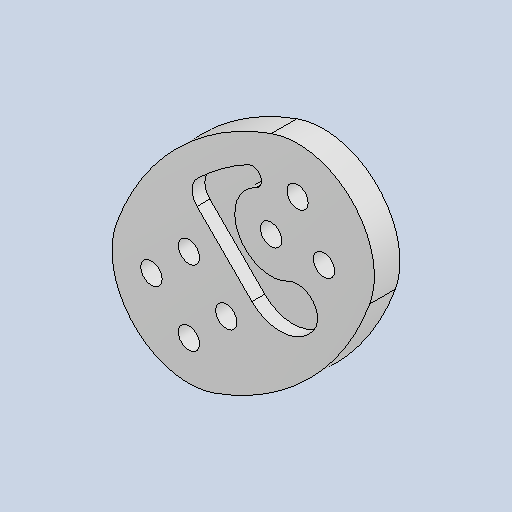
# Autodesk Inventor part: 駆動節
Saved by Autodesk Inventor 2023 (Build 270158000, 158)
## iProperties
Created: 2022-01-08
Part Number: 駆動節
Material: Aluminum 2014-T6
Document SubType Name: Modeling
Designer: acps
Density: 2.78927 g/cm^3
Appearance: Satin
Author: acps
Autodesk Inventor part; units mm, degrees
ref_plane "YZ Plane" through (0, 0, 0) normal (1, 0, 0) x (0, 1, 0)
ref_plane "XZ Plane" through (0, 0, 0) normal (0, 1, 0) x (-1, 0, 0)
ref_plane "XY Plane" through (0, 0, 0) normal (0, 0, 1) x (1, 0, 0)
sketch "Sketch2" plane through (0, 0, 0) normal (0, 0, 1) x (1, 0, 0)
  line L0 (-12.7279, -12.7279) -> (0, 0) construction
  line L1 (-12.7279, -12.7279) -> (-7.4558, -12.7279) construction
  line L2 (-12.7279, -12.7279) -> (0, 0) construction
  line L3 (-17.252, -29.9799) -> (-9.2664, -21.9943) construction
  line L4 (-2.9446, 9.7833) -> (-10.9302, 1.7977) construction
  arc A0 (-21.1882, -9.6582) -> (-9.6582, -21.1882) centre (-12.7279, -12.7279) ccw
  arc A1 (8.4603, -3.0697) -> (-3.0697, 8.4603) centre (0, 0) ccw
  circle A2 centre (-8.3439, -12.7279) radius 1.25
  circle A3 centre (-8.3439, -12.7279) radius 3.1 construction
  circle A4 centre (-12.7279, -8.3439) radius 1.25
  circle A5 centre (-12.7279, -8.3439) radius 3.1 construction
  circle A6 centre (-17.112, -12.7279) radius 1.25
  circle A7 centre (-17.112, -12.7279) radius 3.1 construction
  circle A8 centre (-12.7279, -17.112) radius 1.25
  circle A9 centre (-12.7279, -17.112) radius 3.1 construction
  circle A10 centre (-3.1, -1.7898) radius 1.25
  circle A11 centre (-3.1, -1.7898) radius 3.1 construction
  circle A12 centre (3.1, -1.7898) radius 3.1 construction
  circle A13 centre (3.1, -1.7898) radius 1.25
  circle A14 centre (0, 3.5796) radius 3.1 construction
  circle A15 centre (0, 3.5796) radius 1.25
  arc A16 (-9.6582, -21.1882) -> (8.4603, -3.0697) centre (-19.9758, 7.2478) ccw
  line L5 (1.4142, -14.1421) -> (-6.364, -6.364) construction
  arc A17 (-3.0697, 8.4603) -> (-21.1882, -9.6582) centre (7.2478, -19.9758) ccw
  point P0 (-6.364, -6.364)
  dimension "d34" = 18
  dimension "d35" = 9
  dimension "d36" = 2.5
  dimension "d37" = 6.2
  dimension "d38" = 360
  dimension "d39" = 2.5
  dimension "d40" = 6.2
  dimension "d41" = 360
  dimension "d42" = 11
  dimension "d43" = 45
  constraints: 18 centre point, 14 end point, 9 point on circle, 8 coincident, 8 tangent, 3 symmetric about line, 2 midpoint, 1 horizontal, 1 horizontal alignment, 1 parallel, 1 perpendicular, 1 vertical alignment, 31 other
  measures "d34" distance of L0.start L0.end
  measures "d35" radius of A1
  measures "d36" diameter of A2
  measures "d37" diameter of A3
  measures "d39" diameter of A10
  measures "d40" diameter of A11
  measures "d42" distance of L5.start L5.end
  measures "d43" angle of L1 L0
extrude "Extrusion2" add sketch "Sketch2" along normal blind 3
sketch "Sketch3" plane through (0, 0, 3) normal (0, 0, 1) x (1, 0, 0)
  circle A0 centre (-12.7279, -8.3439) radius 1.25 projected
  circle A1 centre (-8.3439, -12.7279) radius 1.25 projected
  arc A2 (-3.0697, 8.4603) -> (-21.1882, -9.6582) centre (7.2478, -19.9758) ccw projected
  arc A3 (-9.6582, -21.1882) -> (8.4603, -3.0697) centre (-19.9758, 7.2478) ccw projected
  circle A4 centre (-3.1, -1.7898) radius 1.25 projected
  circle A5 centre (3.1, -1.7898) radius 1.25 projected
  circle A6 centre (0, 3.5796) radius 1.25 projected
  arc A7 (-9.6056, 1.4374) -> (-9.622, 1.4245) centre (7.2478, -19.9758) ccw
  circle A8 centre (-12.7279, -8.3439) radius 1.25 projected
  line L0 (-11.844, -7.46) -> (-7.46, -11.844) construction
  arc A9 (1.7167, -9.2445) -> (1.8856, -9.02) centre (-19.9758, 7.2478) ccw
  line L1 (-11.7716, -3.2898) -> (-5.3387, -9.7227)
  line L2 (-5.8854, -0.7722) -> (-0.4613, -6.1962) construction
  arc A10 (1.8856, -9.02) -> (-1.1039, -5.5419) centre (0, -7.6169) ccw
  arc A11 (-5.3387, -9.7227) -> (1.7167, -9.2445) centre (-2.0197, -6.4038) ccw
  circle A12 centre (-8.3439, -12.7279) radius 4.25 construction
  circle A13 centre (-3.1, -1.7898) radius 4.25 construction
  circle A14 centre (3.1, -1.7898) radius 4.25 construction
  circle A15 centre (-12.7279, -8.3439) radius 4.25 construction
  arc A16 (-11.7519, -0.4419) -> (-11.7716, -3.2898) centre (-10.3574, -1.8755) ccw
  arc A17 (-7.1444, 3.1635) -> (-14.769, -3.9189) centre (7.2478, -19.9758) ccw construction
  arc A18 (-4.8412, 2.0872) -> (-1.1039, -5.5419) centre (-3.1, -1.7898) ccw
  arc A19 (-5.7709, 3.9632) -> (-11.7519, -0.4419) centre (7.2478, -19.9758) ccw
  arc A20 (-4.8412, 2.0872) -> (-5.7709, 3.9632) centre (-5.2704, 3.0429) ccw
  circle A21 centre (0, 3.5796) radius 4.25 construction
  point P0 (0, 0)
  point P1 (-1.1039, -5.5419)
  dimension "d46" = 3
  dimension "d49" = 3
  dimension "d52" = 3
  dimension "d53" = 3
  dimension "d54" = 3
  dimension "d55" = 3
  dimension "d56" = 3
  dimension "d59" = 3
  dimension "d60" = 2
  constraints: 22 point on circle, 14 centre point, 13 tangent, 6 concentric, 6 end point, 2 parallel, 5 other
  measures "d46" distance between parallel lines of L0 L1
  measures "d49" radial gap between concentric circles of A3 A9
  measures "d53" radial gap between concentric circles of A4 A13
  measures "d54" radial gap between concentric circles of A5 A14
  measures "d55" radial gap between concentric circles of A0 A15
  measures "d56" radial gap between concentric circles of A2 A17
  measures "d59" radial gap between concentric circles of A6 A21
  measures "d60" radius of A16
extrude "Extrusion3" cut sketch "Sketch3" against normal blind 1.5 contours A19 A20 A18 A10 A9 A11 L1 A16 A7
sketch "sesaku" plane through (0, 0, 3) normal (0, 0, 1) x (1, 0, 0)
  arc A0 (-5.3387, -9.7227) -> (1.7167, -9.2445) centre (-2.0197, -6.4038) ccw projected
  line L0 (-5.3387, -9.7227) -> (-11.7716, -3.2898) projected
  arc A1 (-11.7519, -0.4419) -> (-11.7716, -3.2898) centre (-10.3574, -1.8755) ccw projected
  arc A2 (1.8856, -9.02) -> (-1.1039, -5.5419) centre (0, -7.6169) ccw projected
  arc A3 (1.7167, -9.2445) -> (1.8856, -9.02) centre (-19.9758, 7.2478) ccw projected
  arc A4 (-9.6582, -21.1882) -> (8.4603, -3.0697) centre (-19.9758, 7.2478) ccw projected
  arc A5 (8.4603, -3.0697) -> (-3.0697, 8.4603) centre (0, 0) ccw projected
  arc A6 (-3.0697, 8.4603) -> (-21.1882, -9.6582) centre (7.2478, -19.9758) ccw projected
  arc A7 (-21.1882, -9.6582) -> (-9.6582, -21.1882) centre (-12.7279, -12.7279) ccw projected
  circle A8 centre (0, 3.5796) radius 1.25 projected
  circle A9 centre (3.1, -1.7898) radius 1.25 projected
  circle A10 centre (-3.1, -1.7898) radius 1.25 projected
  circle A11 centre (-12.7279, -17.112) radius 1.25 projected
  circle A12 centre (-17.112, -12.7279) radius 1.25 projected
  circle A13 centre (-12.7279, -8.3439) radius 1.25 projected
  circle A14 centre (-8.3439, -12.7279) radius 1.25 projected
  arc A15 (-5.7709, 3.9632) -> (-11.7519, -0.4419) centre (7.2478, -19.9758) ccw projected
  arc A16 (-4.8412, 2.0872) -> (-5.7709, 3.9632) centre (-5.2704, 3.0429) ccw projected
  arc A17 (-4.8412, 2.0872) -> (-1.1039, -5.5419) centre (-3.1, -1.7898) ccw projected
body "Solid2"
